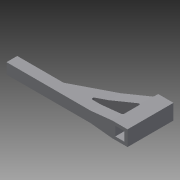
# Autodesk Inventor part: foot_1_2_small
Saved by Autodesk Inventor 2015 SP1 (Build 190203100, 203)
## iProperties
Created: 2015-10-26
Part Number: foot_1_2_small
Material: Generic
Document SubType Name: Modeling
Designer: Alexandre Cherpillod
Density: 1 g/cm^3
Appearance: Default
Author: Alexandre Cherpillod
Autodesk Inventor part; units mm, degrees
ref_plane "YZ Plane" through (0, 0, 0) normal (1, 0, 0) x (0, 1, 0)
ref_plane "XZ Plane" through (0, 0, 0) normal (0, 1, 0) x (-1, 0, 0)
ref_plane "XY Plane" through (0, 0, 0) normal (0, 0, 1) x (1, 0, 0)
sketch "Sketch1" plane through (0, 0, 0) normal (0, 1, 0) x (-1, 0, 0)
  line L0 (0, 0) -> (10, 0)
  line L1 (10, 0) -> (10, -10)
  line L2 (10, -10) -> (0, -10)
  line L3 (0, -10) -> (0, 0)
  line L4 (10, 0) -> (0, -10) construction
  line L5 (10, -10) -> (0, 0) construction
  line L6 (2, -2) -> (8, -2)
  line L7 (8, -2) -> (8, -8)
  line L8 (8, -8) -> (2, -8)
  line L9 (2, -8) -> (2, -2)
  line L10 (2, -2) -> (8, -8) construction
  line L11 (8, -2) -> (2, -8) construction
  point P0 (5, -5)
  dimension "d0" = 10
  dimension "d4" = 6
  dimension "d5" = 6
  constraints: 24 end point, 4 parallel, 4 perpendicular, 3 midpoint, 2 horizontal
  measures "d0" distance of L1.end L2.end
  measures "d4" distance of L7.end L8.end
  measures "d5" distance of L6.end L7.end
extrude "Extrusion1" add sketch "Sketch1" along normal blind 30
sketch "Sketch2" plane through (-10, 0, -10) normal (-1, 0, 0) x (0, 0, 1)
  line L0 (0, 30) -> (10, 30) construction
  line L1 (10, 0) -> (0, 0) projected
  line L2 (10, 0) -> (0, 0) construction
  line L3 (0, 0) -> (0, 7)
  line L4 (0, 7) -> (10, 7)
  line L5 (10, 7) -> (10, 0)
  line L6 (0, 0) -> (0, 30) construction
  line L7 (10, 0) -> (10, 30) construction
  dimension "d8" = 7
  dimension "d9" = 10
  constraints: 8 end point, 2 parallel, 1 horizontal, 1 perpendicular, 1 point on line
  measures "d8" distance of L2.end L3.end
  measures "d9" distance of L3.end L4.end
extrude "Extrusion2" add sketch "Sketch2" along normal blind 69
chamfer "Chamfer1" distance 20 distance2 38.75 1 edges at (-10, 7, -5) measured on face at (-10, 14.6667, -6.6667)
sketch "Sketch3" plane through (0, 0, 0) normal (0, 0, 1) x (1, 0, 0)
  line L0 (-48.75, 7) -> (-79, 7) construction
  line L1 (-10, 27) -> (-10, 30) construction
  line L2 (-9.9219, 6.8486) -> (-33.7809, 6.8486)
  line L3 (-33.7809, 6.8486) -> (-9.9219, 19.163)
  line L4 (-9.9219, 19.163) -> (-9.9219, 6.8486)
  line L5 (-48.75, 7) -> (-10, 27) projected
  point P0 (0, 0)
  dimension "d21" = 7
  constraints: 6 end point, 1 horizontal, 1 parallel, 1 perpendicular
  measures "d21" distance between parallel lines of L5 L3
extrude "Extrusion3" cut sketch "Sketch3" against normal through all
sketch "Sketch6" plane through (0, 0, 0) normal (0, -1, 0) x (1, 0, 0)
  line L0 (-79, -10) -> (-79, 0) construction
  line L1 (-79, -5) -> (0, -5) construction
  line L2 (0, 0) -> (0, -10) construction
  line L3 (-24.2304, -1.5) -> (-79, -1.5)
  line L4 (-79, -1.5) -> (-79, -8.5)
  line L5 (-79, -8.5) -> (-24.2304, -8.5)
  line L6 (-24.2304, -8.5) -> (-24.2304, -1.5) construction
  line L7 (-24.2304, -1.5) -> (-79, -8.5) construction
  line L8 (-79, -1.5) -> (-24.2304, -8.5) construction
  line L9 (-24.2304, -8.5) -> (0, -8.5) construction
  line L10 (-24.2304, -1.5) -> (0, -1.5) construction
  line L11 (-24.2304, -8.5) -> (-10, -10)
  line L12 (0, -10) -> (-10, -10) construction
  line L13 (-24.2304, -1.5) -> (-10, 0)
  line L14 (-10, 0) -> (0, 0) construction
  line L15 (-10, -10) -> (-10, -18.6026)
  line L16 (-10, -18.6026) -> (-95.3433, -18.6026)
  line L17 (-95.3433, -18.6026) -> (-95.3433, 10.4)
  line L18 (-95.3433, 10.4) -> (-10, 10.4)
  line L19 (-10, 10.4) -> (-10, 0)
  point P0 (-51.6152, -5)
  dimension "d22" = 7
  constraints: 32 end point, 7 perpendicular, 5 midpoint, 5 point on line, 2 parallel, 1 horizontal, 1 vertical
  measures "d22" distance of L3.end L4.end
extrude "Extrusion5" cut sketch "Sketch6" against normal through all
hole "Hole1" at (-79, 3.5, -5) direction (1, 0, 0) diameter 4 depth 5
fillet "Fillet1" radius 1 5 edges at (-33.7809, 6.8486, -5) (-9.9219, 6.8486, -5) (-9.9219, 19.163, -5) (-48.75, 7, -5) (-10, 27, -5)
body "Solid1"
